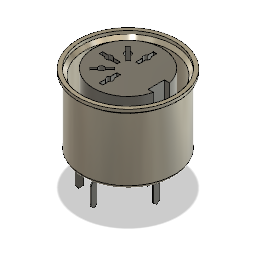
MIDI DIN 5 v7 (Autodesk Fusion 360 design; units mm, degrees)
Autodesk Fusion 360 part; units mm, degrees
sketch "Sketch1" plane through (0, 0, 0) normal (0, 1, 0) x (1, 0, 0)
  circle A0 centre (0, 0) radius 8
  circle A1 centre (0, 0) radius 7.4
  circle A2 centre (0, 0) radius 5.5
  line L0 (4.5, 0) -> (4.5, 1.3)
  line L1 (4.5, 0) -> (4.5, -1.3)
  line L2 (4.5, 1.3) -> (5.3442, 1.3)
  line L3 (4.5, -1.3) -> (5.3442, -1.3)
  circle A3 centre (0, 0) radius 6.8
sketch "Sketch2" plane through (0, 0, 0) normal (0, 1, 0) x (-1, 0, 0)
  circle A0 centre (-7.8928, -5.2339) radius 1
  circle A1 centre (-10.7389, -2.8014) radius 1
  circle A2 centre (-10.239, -4.8215) radius 1
  circle A3 centre (0, 0) radius 5.5
  circle A4 centre (0, 0) radius 5.0572
  circle A5 centre (0, 0) radius 4.7935
  line L0 (-10.7389, -10.0009) -> (-10.7389, 10.3886)
  circle A6 centre (0, 0) radius 8
sketch "Sketch3" plane through (0, 0, 0) normal (0, 1, 0) x (1, 0, 0)
  line L0 (-4.7886, 0.2438) -> (-1.7886, 0.2438)
  line L1 (-1.7886, 0.2438) -> (-1.7886, -0.2562)
  line L2 (-1.7886, -0.2562) -> (-4.7886, -0.2562)
  line L3 (-4.7886, -0.2562) -> (-4.7886, 0.2438)
  line L4 (10.7389, 10.0009) -> (10.7389, -10.3886)
  line L5 (10, 0) -> (-13, 0)
  line L6 (0, 0) -> (-7.0711, -7.0711)
  line L7 (0, 0) -> (10, 0) construction
  line L8 (0, 0) -> (-7.0711, 7.0711)
  circle A0 centre (0, 0) radius 1.8068
  dimension "d13" = 3
  dimension "d14" = 0.5
  dimension "d17" = 135
  dimension "d18" = 10
  dimension "d19" = 10
  measures "d17" angle of L6 L7
  measures "d18" distance of L6.start
  measures "d19" distance of L6.start
sketch "Sketch4" plane through (0, 15.8, 0) normal (0, 1, 0) x (-1, 0, 0)
  line L0 (-4.5, 1.3) -> (-4.5, -1.3)
  line L1 (-4.5, -1.3) -> (-5.3442, -1.3)
  arc A0 (-5.3442, -1.3) -> (-5.3442, 1.3) centre (0, 0) ccw
  line L2 (-5.3442, 1.3) -> (-4.5, 1.3)
  line L3 (0, 13) -> (0, -9)
sketch "Sketch5" plane through (0, 0, 0) normal (0, 0, 1) x (1, 0, 0)
  line L0 (5.3442, 15.8) -> (-5.5, 15.8)
  line L1 (0, -15) -> (0, 25)
  line L2 (15, 0) -> (-15, 0)
sketch "Sketch6" plane through (0, 0, 0) normal (0, 1, 0) x (1, 0, 0)
  line L0 (-1.5, 0.25) -> (-4.3, 0.25)
  line L1 (-4.3, 0.25) -> (-4.3, -0.25)
  line L2 (-4.3, -0.25) -> (-1.5, -0.25)
  line L3 (-1.5, -0.25) -> (-1.5, 0.25)
  line L4 (-4.3, 0.25) -> (-4.3, -0.25)
  line L5 (-4.3, 0) -> (-4.36, 0)
  line L6 (-3.0406, -3.0406) -> (-3.083, -3.083)
  line L7 (-3.2173, -2.8638) -> (-2.8638, -3.2173)
  line L8 (-0.8839, -1.2374) -> (-1.2374, -0.8839)
  line L9 (-2.8638, -3.2173) -> (-0.8839, -1.2374)
  line L10 (-3.2173, -2.8638) -> (-2.8638, -3.2173)
  line L11 (-1.2374, -0.8839) -> (-3.2173, -2.8638)
  line L12 (-0.2781, 1.5) -> (0.2781, 1.5)
  line L13 (0.2781, 1.5) -> (0.2781, 4.3)
  line L14 (0.2781, 4.3) -> (-0.2781, 4.3)
  line L15 (0, 4.3) -> (0, 4.36)
  line L16 (0.2781, 4.3) -> (-0.2781, 4.3)
  line L17 (-0.2781, 4.3) -> (-0.2781, 1.5)
  circle A0 centre (-3, 0) radius 0.5
  circle A1 centre (-2.052, -2.052) radius 0.5
  circle A2 centre (0, 2.902) radius 0.5
  line L18 (-2.8638, 3.2173) -> (-3.2173, 2.8638)
  line L19 (-2.8638, 3.2173) -> (-3.2173, 2.8638)
  line L20 (-0.8839, 1.2374) -> (-2.8638, 3.2173)
  line L21 (-1.2374, 0.8839) -> (-0.8839, 1.2374)
  line L22 (-3.2173, 2.8638) -> (-1.2374, 0.8839)
  line L23 (-3.0406, 3.0406) -> (-3.083, 3.083)
  circle A3 centre (-2.1213, 2.1213) radius 0.5
  circle A4 centre (0, -3) radius 0.5
  line L24 (0, -4.3) -> (0, -4.36)
  line L25 (-0.25, -4.3) -> (0.25, -4.3)
  line L26 (0.25, -1.5) -> (-0.25, -1.5)
  line L27 (0.25, -4.3) -> (0.25, -1.5)
  line L28 (-0.25, -4.3) -> (0.25, -4.3)
  line L29 (-0.25, -1.5) -> (-0.25, -4.3)
  dimension "d20" = 2.8
  dimension "d22" = 2.8
  dimension "d25" = 2.8
  dimension "d26" = 1
  dimension "d27" = 1
  dimension "d30" = 1
  dimension "d34" = 2.8
  dimension "d35" = 1
  dimension "d36" = 2.8
  dimension "d37" = 1
  measures "d26" diameter of A0
  measures "d27" diameter of A1
  measures "d30" diameter of A2
  measures "d35" diameter of A3
  measures "d37" diameter of A4
sketch "Sketch7" plane through (0, 0, 0) normal (0, 1, 0) x (1, 0, 0)
sketch "Sketch8" plane through (0, 0, 0) normal (0, 1, 0) x (1, 0, 0)
  circle A0 centre (0, -2.902) radius 0.5
  dimension "d31" = 1
  measures "d31" diameter of A0
extrude "Extrude2" add sketch "Sketch1" along normal blind 10 contours A2 L0 L1 L2 L3 picked at (2.4488, 2.1818) makes body 1
sketch "Sketch9" plane through (0, 0, 0) normal (0, 1, 0) x (-1, 0, 0)
extrude "Extrude3" cut sketch "Sketch6" along normal blind 100 bodies 1
sketch "Sketch10" plane through (0, 0, 0) normal (0, 0, 1) x (1, 0, 0)
  line L0 (8, 0) -> (-8, 0)
  line L1 (-8, 0) -> (-8, 0.5)
  line L2 (-8, 0.5) -> (-7.4, 1)
  line L3 (-7.4, 1) -> (-7.4, 11)
  arc A0 (-7, 11.5) -> (-7.4, 11) centre (-6.8875, 11) ccw
  arc A1 (-6.9045, 11.5) -> (-7.5156, 11.2783) centre (-6.8875, 10.5) ccw
  arc A2 (7, 11.5) -> (7.4, 11) centre (6.8875, 11) cw
  line L4 (-6.9045, 11.5) -> (7, 11.5)
  line L5 (8, 0) -> (8, 0.5)
  line L6 (8, 1) -> (-8, 1)
  line L7 (8, 0.5) -> (7.4, 1)
  line L8 (7.4, 1) -> (7.4, 11)
  line L9 (-6.8875, 10.5) -> (-6.8875, 1)
  line L10 (-7.4, 0.5) -> (-7.4, 0)
  arc A3 (-6.4895, 10.9976) -> (-6.8875, 10.5) centre (-6.3769, 10.4996) ccw
  line L11 (-7.4, 0.5) -> (-6.8875, 1)
  line L12 (-6.4895, 10.9976) -> (0, 11)
  line L13 (0, -0.5) -> (0, -2)
  line L14 (7.4, 0.5) -> (7.4, 0)
  line L15 (7.4, 0.5) -> (6.8875, 1)
  line L16 (6.8875, 10.5) -> (6.8875, 1)
  arc A4 (6.4895, 10.9976) -> (6.8875, 10.5) centre (6.3769, 10.4996) cw
  line L17 (6.4895, 10.9976) -> (0, 11)
  line L18 (0, 11) -> (0, 11.5)
revolve "Revolve1" add sketch "Sketch10" angle 360 about axis through (0, -0.5, 0) along (0, -1, 0) separate body contours L0 L1 L2 L6 L10 L11 | L3 A0 A1 L4 L6 L9 A3 L12 L18 makes body 2
sketch "Sketch11" plane through (0, 0, 0) normal (0, 0, 1) x (1, 0, 0)
  line L0 (-10, 0) -> (-10, 15.8) construction
  line L1 (-10, 15.8) -> (14, 15.8) construction
  line L2 (6.9045, 11.5) -> (-6.9045, 11.5)
  line L3 (7.0452, 11.4876) -> (-7.0452, 11.4876)
  line L4 (6.8838, 11.5) -> (6.8838, 12.5)
  line L5 (6.8838, 12.5) -> (-6.9, 12.5)
  line L6 (-6.9, 12.5) -> (-6.9045, 11.5)
  line L7 (0, -2.5) -> (0, 22.5) construction
  line L8 (0, 15.8) -> (-5.5, 15.8) construction
  dimension "d48" = 15.8
  dimension "d49" = 24
  dimension "d50" = 5.5
sketch "Sketch12" plane through (0, 0, 0) normal (0, 1, 0) x (1, 0, 0)
  circle A0 centre (0, 0) radius 5.5
  line L0 (0, 0) -> (-10, -10) construction
  line L1 (0, 0) -> (-10, 10) construction
  circle A1 centre (-5.5, 0) radius 0.7
  circle A2 centre (-3.8891, -3.8891) radius 0.7
  line L2 (6.8838, 0) -> (-6.9, 0) construction
  line L3 (0, -10) -> (0, 10) construction
  circle A3 centre (0, -5.5) radius 0.7
  circle A4 centre (-3.8891, 3.8891) radius 0.7
  circle A5 centre (0, 5.5) radius 0.7
  line L4 (0, 5.5) -> (4.5, 5.5) construction
  line L5 (4.5, 5.5) -> (4.5, -5.5) construction
  circle A6 centre (4.5, 0) radius 0.7
  dimension "d51" = 11
  dimension "d52" = 1.4
  dimension "d53" = 1.4
  dimension "d54" = 1.4
  dimension "d55" = 1.4
  dimension "d56" = 1.4
  dimension "d57" = 4.5
  dimension "d58" = 11
  dimension "d59" = 1.4
  measures "d51" diameter of A0
  measures "d52" diameter of A1
  measures "d53" diameter of A2
  measures "d54" diameter of A3
  measures "d55" diameter of A4
  measures "d56" diameter of A5
  measures "d59" diameter of A6
move_body "Move3" bodies 1 2 to x (1, 0, 0) y (0, -1, 0) z (0, 0, -1) at (0, 0, 0)
move_body "Move4" bodies 1 2 to x (1, 0, 0) y (0, 1, 0) z (0, 0, 1) at (0, 15.8, 0)
extrude "Extrude7" add sketch "Sketch12" along normal blind 1 separate body contours A0 A1 A2 A3 A4 A5 | A0 A5 | A0 A3 | A0 A4 | A0 A2 | A0 A1 | A6 picked at (-0.0167, 5.264) picked at (0.0167, -5.264) picked at (-3.7108, 3.7335) picked at (-3.7108, -3.7335) picked at (-5.2634, 0) makes body 3
move_body "Move5" bodies 3 to x (1, 0, 0) y (0, 1, 0) z (0, 0, 1) at (0, 3.3, 0)
sketch "Sketch13" plane through (0, 0, 0) normal (1, 0, 0) x (0, 0, -1)
  line L0 (-7.0452, 4.3124) -> (7.0452, 4.3124) construction
  line L1 (-6.9045, 4.3) -> (6.9045, 4.3) construction
  line L2 (-5.5, 0) -> (-5.5, 4.3124) construction
  line L3 (5.5, 3.3) -> (-5.5, 3.3) construction
  line L4 (-5, 0) -> (-5, 3.3) construction
  line L5 (-6, 0) -> (-6, 4.3) construction
  line L6 (-7.5, 2.5) -> (6.5, 2.5) construction
  line L7 (-5.5, 3.3) -> (-7.5, 3.3) construction
  line L8 (-7.5, -0.7) -> (6, -0.7) construction
  line L9 (-5.5, 0) -> (-5.5, -0.7) construction
  line L10 (-5.5, -0.7) -> (-5, -0.7)
  line L11 (-6, 2.5) -> (-5.5, 3.3)
  line L12 (-6, 2.5) -> (-6, 0)
  line L13 (-5.5, -0.7) -> (-5.6, -0.7)
  line L14 (-5.5, -0.7) -> (-5.4, -0.7)
  line L15 (-5, 0) -> (-5, -1.5) construction
  line L16 (-5.4, -0.7) -> (-5, -0.3)
  line L17 (-5, -0.3) -> (-5, 2.5)
  line L18 (-5, 2.5) -> (-4.5003, 2.5)
  line L19 (-4.5003, 2.5) -> (-4.5003, 3.3)
  line L20 (-4.5003, 3.3) -> (-5.5, 3.3)
  line L21 (-6, 0) -> (-6, -0.7) construction
  line L22 (-5.6, -0.7) -> (-6, -0.3)
  line L23 (-6, -0.3) -> (-6, 0)
  dimension "d69" = 4
  dimension "d70" = 0.5
extrude "Extrude8" add sketch "Sketch13" along normal blind 0.1 and the other way blind 0.1 separate body makes body 4
copy_body "CopyPasteBodies1" bodies 4 makes body 5
move_body "Move6" bodies 5 to x (0.707107, 0, 0.707107) y (0, 1, 0) z (-0.707107, 0, 0.707107) at (0, 0, 0)
copy_body "CopyPasteBodies2" bodies 5 makes body 6
move_body "Move7" bodies 6 to x (0.707107, 0, 0.707107) y (0, 1, 0) z (-0.707107, 0, 0.707107) at (0, 0, 0)
copy_body "CopyPasteBodies3" bodies 6 makes body 7
move_body "Move8" bodies 7 to x (0.707107, 0, 0.707107) y (0, 1, 0) z (-0.707107, 0, 0.707107) at (0, 0, 0)
copy_body "CopyPasteBodies4" bodies 7 makes body 8
move_body "Move9" bodies 8 to x (0.707107, 0, 0.707107) y (0, 1, 0) z (-0.707107, 0, 0.707107) at (0, 0, 0)
copy_body "CopyPasteBodies5" bodies 8 makes body 9
move_body "Move10" bodies 9 to x (0, 0, 1) y (0, 1, 0) z (-1, 0, 0) at (0, 0, 0)
move_body "Move11" bodies 9 to x (1, 0, 0) y (0, 1, 0) z (0, 0, 1) at (-0.8, 0, 0)
sketch "Sketch14" plane through (0, 0, 0) normal (0, 1, 0) x (-1, 0, 0)
sketch "Sketch16" plane through (0, 0, 0) normal (1, 0, 0) x (0, 0, -1)
  line L0 (-0.1, 3.3) -> (0.1, 3.3)
  line L1 (-0.1, 2.5) -> (-0.1, 3.3) construction
  line L2 (0, 3.3) -> (-2, 3.3)
  line L3 (-2, 2.5) -> (-0.5, 2.5)
  line L4 (-0.5, 2.5) -> (-0.5, -0.3)
  line L5 (-0.5, -0.3) -> (-0.1, -0.7)
  line L6 (-0.1, -0.7) -> (0.1, -0.7)
  line L7 (0.1, -0.7) -> (0.5, -0.3)
  line L8 (0.5, -0.3) -> (0.5, 2.5)
  line L9 (0.5, 2.5) -> (2, 2.5)
  line L10 (2, 2.5) -> (2, 3.3)
  line L11 (2, 3.3) -> (0.1, 3.3)
  line L12 (-2, 3.3) -> (-2, 2.5)
  line L13 (-1.5, 3.5) -> (-1.5, 2)
  line L14 (1.5, 3.5) -> (1.5, 1.9896)
extrude "Extrude9" add sketch "Sketch16" along normal mid plane 0.2 separate body contours L0 L2 L3 L4 L5 L6 L7 L8 L9 L11 L13 L14 makes body 10
move_body "Move12" bodies 10 to x (1, 0, 0) y (0, 1, 0) z (0, 0, 1) at (-5.5, 0, 0)
move_body "Move13" bodies 10 to x (1, 0, 0) y (0, 1, 0) z (0, 0, 1) at (10, 0, 0)
hidden bodies 9
named bodies: "PIN", "PIN (1)", "PIN (1) (1)", "PIN (1) (1) (1)", "PIN (1) (1) (1) (1)", "PIN (1) (1) (1) (1) (1)"
